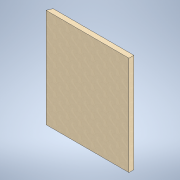
# Autodesk Inventor part: PlatteAussenEineSeite
Saved by Autodesk Inventor 2020.3 (Build 243373010, 373A)
## iProperties
Created: 2021-02-12
Part Number: PlatteAussenEineSeite
Material: Generisch
Document SubType Name: Modeling
Designer: Stefan
Density: 1 g/cm^3
Appearance: Pappel
Author: Stefan
Autodesk Inventor part; units mm, degrees
ref_plane "YZ Plane" through (0, 0, 0) normal (1, 0, 0) x (0, 1, 0)
ref_plane "XZ Plane" through (0, 0, 0) normal (0, 1, 0) x (-1, 0, 0)
ref_plane "XY Plane" through (0, 0, 0) normal (0, 0, 1) x (1, 0, 0)
sketch "Skizze1" plane through (0, 0, 0) normal (0, 0, 1) x (1, 0, 0)
  line L0 (-149.1768, 16.7418) -> (13.9312, 16.7418)
  line L1 (13.9312, 16.7418) -> (13.9312, -183.2582)
  line L2 (13.9312, -183.2582) -> (-149.1768, -183.2582)
  line L3 (-149.1768, -183.2582) -> (-149.1768, 16.7418)
  point P0 (0, 0)
  dimension "d0" = 200
  dimension "d1" = 163.108
  constraints: 8 end point, 2 parallel, 1 horizontal, 1 perpendicular
  measures "d0" distance of L0.end L1.end
  measures "d1" distance of L0.start L0.end
extrude "Extrusion1" add sketch "Skizze1" along normal blind 10
sketch "Skizze3" plane through (-149.1768, -183.2582, 0) normal (0, -1, 0) x (1, 0, 0)
  line L0 (0, 0) -> (163.108, 0) projected
  line L1 (0, 0) -> (0, 10) projected
  line L2 (0, 0) -> (0, 10)
  line L3 (0, 0) -> (-4.1421, 10)
  line L4 (0, 10) -> (163.108, 10) projected
  line L5 (0, 10) -> (-4.1421, 10)
  point P0 (149.1768, 0)
  dimension "d4" = 22.5
  constraints: 6 end point, 1 collinear, 1 horizontal
  measures "d4" angle of L3 L1
extrude "Extrusion2" add sketch "Skizze3" against normal up to surface (200 mm away)
